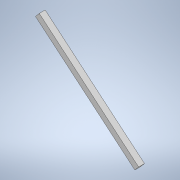
# Autodesk Inventor part: newPullyV03
Saved by Autodesk Inventor 2020.2 (Build 242310000, 310)
## iProperties
Created: 2020-02-22
Part Number: newPullyV03
Material: Generic
Document SubType Name: Modeling
Designer: robst
Density: 1 g/cm^3
Appearance: Default
Author: robst
Autodesk Inventor part; units mm, degrees
ref_plane "YZ Plane" through (0, 0, 0) normal (1, 0, 0) x (0, 1, 0)
ref_plane "XZ Plane" through (0, 0, 0) normal (0, 1, 0) x (-1, 0, 0)
ref_plane "XY Plane" through (0, 0, 0) normal (0, 0, 1) x (1, 0, 0)
sketch "Sketch1" plane through (0, 0, 0) normal (0, 0, 1) x (1, 0, 0)
  line L0 (-351.8656, 461.0371) -> (76.2, 101.8473)
  line L1 (76.2, 135.0047) -> (-335.5388, 480.4946)
  line L2 (-335.5388, 480.4946) -> (-351.8656, 461.0371)
  line L3 (0, 0) -> (0, 391.6762) construction
  line L4 (76.2, 135.0047) -> (76.2, 101.8473)
  line L5 (76.2, 135.0047) -> (92.5268, 121.3049)
  line L6 (76.2, 101.8473) -> (92.5268, 121.3049)
  dimension "d29" = 76.2
  dimension "d30" = 558.8
  constraints: 14 end point, 2 vertical, 1 parallel, 1 perpendicular
  measures "d29" distance between parallel lines of L4 L3
  measures "d30" distance of L0.start L0.end
extrude "Extrusion2" add sketch "Sketch1" along normal mid plane 25.4
body "Solid2"
